Autodesk Fusion 360 part; units mm, degrees
(part 2 of 3)
  line L895 (-90.4101, 0.75) -> (-90.4101, -0.75)
  line L896 (-91.5158, -0.75) -> (-91.5158, 0.75)
  line L897 (-84.4232, -19.1686) -> (-85.7222, -18.4186)
  line L898 (-101.5213, 0.75) -> (-101.5213, -0.75)
  line L899 (-80.3306, -0.75) -> (-80.3306, 0.75)
  line L900 (-94.1139, 0.75) -> (-94.1139, -0.75)
  line L901 (-87.463, -11.6036) -> (-86.1639, -10.8536)
  line L902 (-81.6296, 1.5) -> (-82.9287, 0.75)
  line L903 (-100.2222, 1.5) -> (-101.5213, 0.75)
  line L904 (-121.5343, -20.6686) -> (-121.5343, -19.1686)
  line L905 (-97.8176, 0.75) -> (-97.8176, -0.75)
  line L906 (-72.6481, -11.6036) -> (-71.3491, -10.8536)
  line L907 (-85.3333, 1.5) -> (-86.6324, 0.75)
  line L908 (-63.1111, 1.5) -> (-64.4101, 0.75)
  line L909 (-122.299, -17.4932) -> (-121, -18.2432)
  line L910 (-95.2195, -0.75) -> (-95.2195, 0.75)
  line L911 (-84.0343, 0.75) -> (-85.3333, 1.5)
  line L912 (-96.5185, 1.5) -> (-97.8176, 0.75)
  line L913 (-70.2435, -10.8536) -> (-68.9444, -11.6036)
  line L914 (-80.3306, 0.75) -> (-81.6296, 1.5)
  line L915 (-76.6269, 0.75) -> (-77.9259, 1.5)
  line L916 (-59.3333, 1.5) -> (-60.6324, 0.75)
  line L917 (-40.8148, 1.5) -> (-42.1139, 0.75)
  line L918 (-51.6509, -10.8536) -> (-50.3519, -11.6036)
  line L919 (-107.3546, -10.8536) -> (-106.0556, -11.6036)
  line L920 (-46.9232, 0.75) -> (-48.2222, 1.5)
  line L921 (-55.6296, 1.5) -> (-56.9287, 0.75)
  line L922 (-61.8121, -0.75) -> (-61.8121, 0.75)
  line L923 (-48.2222, 1.5) -> (-49.5213, 0.75)
  line L924 (-64.4101, 0.75) -> (-64.4101, -0.75)
  line L925 (-50.6269, -0.75) -> (-50.6269, 0.75)
  line L926 (-69.2195, -0.75) -> (-69.2195, 0.75)
  line L927 (-62.762, -10.8536) -> (-61.463, -11.6036)
  line L928 (-71.8176, 0.75) -> (-71.8176, -0.75)
  line L929 (-117.8306, -19.1686) -> (-119.1296, -18.4186)
  line L930 (-120.4287, -20.6686) -> (-119.1296, -21.4186)
  line L931 (-122.299, -15.9932) -> (-122.299, -17.4932)
  line L932 (-119.1296, -21.4186) -> (-117.8306, -20.6686)
  line L933 (-106.3306, -0.75) -> (-106.3306, 0.75)
  line L934 (-119.701, -17.4932) -> (-119.701, -15.9932)
  line L935 (-53.225, 0.75) -> (-53.225, -0.75)
  line L936 (-117.8306, -20.6686) -> (-117.8306, -19.1686)
  line L937 (-120.4287, -19.1686) -> (-120.4287, -20.6686)
  line L938 (-54.3306, -0.75) -> (-54.3306, 0.75)
  line L939 (-109.7593, -11.6036) -> (-108.4602, -10.8536)
  line L940 (-92.8148, 1.5) -> (-94.1139, 0.75)
  line L941 (-68.9444, -11.6036) -> (-67.6454, -10.8536)
  line L942 (-37.1111, 1.5) -> (-38.4101, 0.75)
  line L943 (-98.6481, -11.6036) -> (-97.3491, -10.8536)
  line L944 (-98.9232, 0.75) -> (-100.2222, 1.5)
  line L945 (-87.8121, 0.75) -> (-89.1111, 1.5)
  line L946 (-95.2195, 0.75) -> (-96.5185, 1.5)
  line L947 (-39.5158, 0.75) -> (-40.8148, 1.5)
  line L948 (-92.4657, -10.8536) -> (-91.1667, -11.6036)
  line L949 (-54.3306, 0.75) -> (-55.6296, 1.5)
  line L950 (-83.7593, -11.6036) -> (-82.4602, -10.8536)
  line L951 (-91.5158, 0.75) -> (-92.8148, 1.5)
  line L952 (-44.5185, 1.5) -> (-45.8176, 0.75)
  line L953 (-94.9444, -11.6036) -> (-93.6454, -10.8536)
  line L954 (-99.9472, -10.8536) -> (-98.6481, -11.6036)
  line L955 (-87.0213, -20.6686) -> (-85.7222, -21.4186)
  line L956 (-73.9472, -10.8536) -> (-72.6481, -11.6036)
  line L957 (-89.1111, -1.5) -> (-87.8121, -0.75)
  line L958 (-47.9472, -10.8536) -> (-46.6481, -11.6036)
  line L959 (-70.5185, 1.5) -> (-71.8176, 0.75)
  line L960 (-50.6269, 0.75) -> (-51.9259, 1.5)
  line L961 (-77.6509, -10.8536) -> (-76.3519, -11.6036)
  line L962 (-35.8121, 0.75) -> (-37.1111, 1.5)
  line L963 (-66.8148, 1.5) -> (-68.1139, 0.75)
  line L964 (-79.6139, -19.1686) -> (-79.6139, -20.6686)
  line L965 (-66.4657, -10.8536) -> (-65.1667, -11.6036)
  line L966 (-44.2435, -10.8536) -> (-42.9444, -11.6036)
  line L967 (-72.9232, 0.75) -> (-74.2222, 1.5)
  line L968 (-107.6296, 1.5) -> (-108.9287, 0.75)
  line L969 (-54.0556, -11.6036) -> (-52.7565, -10.8536)
  line L970 (-91.1667, -11.6036) -> (-89.8676, -10.8536)
  line L971 (-65.1667, -11.6036) -> (-63.8676, -10.8536)
  line L972 (-77.0158, -19.1686) -> (-78.3148, -18.4186)
  line L973 (-84.4232, -20.6686) -> (-84.4232, -19.1686)
  line L974 (-61.8121, 0.75) -> (-63.1111, 1.5)
  line L975 (-74.2222, 1.5) -> (-75.5213, 0.75)
  line L976 (-58.0343, 0.75) -> (-59.3333, 1.5)
  line L977 (-69.2195, 0.75) -> (-70.5185, 1.5)
  line L978 (-51.9259, 1.5) -> (-53.225, 0.75)
  line L979 (-85.0583, -10.8536) -> (-83.7593, -11.6036)
  line L980 (-42.9444, -11.6036) -> (-41.6454, -10.8536)
  line L981 (-111.0583, -10.8536) -> (-109.7593, -11.6036)
  line L982 (-106.3306, 0.75) -> (-107.6296, 1.5)
  line L983 (-103.9259, 1.5) -> (-105.225, 0.75)
  line L984 (-50.3519, -11.6036) -> (-49.0528, -10.8536)
  line L985 (-57.7593, -11.6036) -> (-56.4602, -10.8536)
  line L986 (-43.2195, 0.75) -> (-44.5185, 1.5)
  line L987 (-102.6269, 0.75) -> (-103.9259, 1.5)
  line L988 (-55.3546, -10.8536) -> (-54.0556, -11.6036)
  line L989 (-76.3519, -11.6036) -> (-75.0528, -10.8536)
  line L990 (-78.3148, -18.4186) -> (-79.6139, -19.1686)
  line L991 (-106.0556, -11.6036) -> (-104.7565, -10.8536)
  line L992 (-88.762, -10.8536) -> (-87.463, -11.6036)
  line L993 (-103.6509, -10.8536) -> (-102.3519, -11.6036)
  line L994 (-59.0583, -10.8536) -> (-57.7593, -11.6036)
  line L995 (-89.1667, -8.1395) -> (-87.8676, -7.3895)
  line L996 (-65.5158, 0.75) -> (-66.8148, 1.5)
  line L997 (-96.2435, -10.8536) -> (-94.9444, -11.6036)
  line L998 (-77.9259, 1.5) -> (-79.225, 0.75)
  line L999 (-102.3519, -11.6036) -> (-101.0528, -10.8536)
  line L1000 (-80.0556, -11.6036) -> (-78.7565, -10.8536)
  line L1001 (-89.1111, 1.5) -> (-90.4101, 0.75)
  line L1002 (-46.6481, -11.6036) -> (-45.3491, -10.8536)
  line L1003 (-61.463, -11.6036) -> (-60.1639, -10.8536)
  line L1004 (-81.3546, -10.8536) -> (-80.0556, -11.6036)
  line L1005 (-96.299, -17.4932) -> (-95, -18.2432)
  line L1006 (-95, -15.2432) -> (-96.299, -15.9932)
  line L1007 (-83.3176, -20.6686) -> (-82.0185, -21.4186)
  line L1008 (-87.8676, -5.8895) -> (-89.1667, -5.1395)
  line L1009 (-99.0528, -5.8895) -> (-100.3519, -5.1395)
  line L1010 (-87.5926, -15.2432) -> (-88.8916, -15.9932)
  line L1011 (-179.9101, -19.1686) -> (-179.9101, -20.6686)
  line L1012 (-177.3121, -19.1686) -> (-178.6111, -18.4186)
  line L1013 (-173.5343, -19.1686) -> (-174.8333, -18.4186)
  line L1014 (-176.1324, -19.1686) -> (-176.1324, -20.6686)
  line L1015 (-173.5343, -20.6686) -> (-173.5343, -19.1686)
  line L1016 (-174.8333, -18.4186) -> (-176.1324, -19.1686)
  line L1017 (-178.6111, -21.4186) -> (-177.3121, -20.6686)
  line L1018 (-181.0158, -19.1686) -> (-182.3148, -18.4186)
  line L1019 (-184.7195, -19.1686) -> (-186.0185, -18.4186)
  line L1020 (-187.3176, -20.6686) -> (-186.0185, -21.4186)
  line L1021 (-188.4232, -19.1686) -> (-189.7222, -18.4186)
  line L1022 (-181.7805, -15.9932) -> (-181.7805, -17.4932)
  line L1023 (-180.8861, -12.5291) -> (-182.1852, -11.7791)
  line L1024 (-184.5899, -14.0291) -> (-184.5899, -12.5291)
  line L1025 (-186.5899, -15.9932) -> (-187.8889, -15.2432)
  line L1026 (-183.4842, -14.0291) -> (-182.1852, -14.7791)
  line L1027 (-184.1852, -15.2432) -> (-185.4842, -15.9932)
  line L1028 (-187.1879, -12.5291) -> (-187.1879, -14.0291)
  line L1029 (-183.4842, -12.5291) -> (-183.4842, -14.0291)
  line L1030 (-185.4842, -17.4932) -> (-184.1852, -18.2432)
  line L1031 (-185.8889, -11.7791) -> (-187.1879, -12.5291)
  line L1032 (-187.8889, -15.2432) -> (-189.1879, -15.9932)
  line L1033 (-166.1269, -20.6686) -> (-166.1269, -19.1686)
  line L1034 (-169.8306, -19.1686) -> (-171.1296, -18.4186)
  line L1035 (-171.1296, -21.4186) -> (-169.8306, -20.6686)
  line L1036 (-168.725, -20.6686) -> (-167.4259, -21.4186)
  line L1037 (-172.4287, -19.1686) -> (-172.4287, -20.6686)
  line L1038 (-172.4287, -20.6686) -> (-171.1296, -21.4186)
  line L1039 (-167.4259, -21.4186) -> (-166.1269, -20.6686)
  line L1040 (-168.725, -19.1686) -> (-168.725, -20.6686)
  line L1041 (-171.1296, -18.4186) -> (-172.4287, -19.1686)
  line L1042 (-167.4259, -18.4186) -> (-168.725, -19.1686)
  line L1043 (-179.9101, -20.6686) -> (-178.6111, -21.4186)
  line L1044 (-174.8333, -21.4186) -> (-173.5343, -20.6686)
  line L1045 (-177.3121, -20.6686) -> (-177.3121, -19.1686)
  line L1046 (-173.4787, -14.0291) -> (-173.4787, -12.5291)
  line L1047 (-174.7778, -11.7791) -> (-176.0768, -12.5291)
  line L1048 (-175.4787, -15.9932) -> (-176.7778, -15.2432)
  line L1049 (-179.1824, -15.9932) -> (-180.4815, -15.2432)
  line L1050 (-176.7778, -15.2432) -> (-178.0768, -15.9932)
  line L1051 (-174.7778, -14.7791) -> (-173.4787, -14.0291)
  line L1052 (-179.1824, -17.4932) -> (-179.1824, -15.9932)
  line L1053 (-173.4787, -12.5291) -> (-174.7778, -11.7791)
  line L1054 (-179.7805, -12.5291) -> (-179.7805, -14.0291)
  line L1055 (-176.7778, -18.2432) -> (-175.4787, -17.4932)
  line L1056 (-177.1824, -12.5291) -> (-178.4815, -11.7791)
  line L1057 (-178.4815, -14.7791) -> (-177.1824, -14.0291)
  line L1058 (-189.463, -8.1395) -> (-188.1639, -7.3895)
  line L1059 (-176.0768, -12.5291) -> (-176.0768, -14.0291)
  line L1060 (-182.1852, -14.7791) -> (-180.8861, -14.0291)
  line L1061 (-185.4842, -15.9932) -> (-185.4842, -17.4932)
  line L1062 (-182.8861, -17.4932) -> (-182.8861, -15.9932)
  line L1063 (-184.1852, -18.2432) -> (-182.8861, -17.4932)
  line L1064 (-182.1852, -11.7791) -> (-183.4842, -12.5291)
  line L1065 (-189.1879, -15.9932) -> (-189.1879, -17.4932)
  line L1066 (-189.1879, -17.4932) -> (-187.8889, -18.2432)
  line L1067 (-178.6111, -18.4186) -> (-179.9101, -19.1686)
  line L1068 (-176.1324, -20.6686) -> (-174.8333, -21.4186)
  line L1069 (-168.5953, -12.5291) -> (-168.5953, -14.0291)
  line L1070 (-169.701, -14.0291) -> (-169.701, -12.5291)
  line L1071 (-166.8916, -15.9932) -> (-166.8916, -17.4932)
  line L1072 (-169.2963, -18.2432) -> (-167.9973, -17.4932)
  line L1073 (-171, -11.7791) -> (-172.299, -12.5291)
  line L1074 (-167.9973, -15.9932) -> (-169.2963, -15.2432)
  line L1075 (-169.701, -12.5291) -> (-171, -11.7791)
  line L1076 (-170.5953, -15.9932) -> (-170.5953, -17.4932)
  line L1077 (-169.2963, -15.2432) -> (-170.5953, -15.9932)
  line L1078 (-172.299, -12.5291) -> (-172.299, -14.0291)
  line L1079 (-189.5926, -14.7791) -> (-188.2936, -14.0291)
  line L1080 (-167.2963, -11.7791) -> (-168.5953, -12.5291)
  line L1081 (-170.5953, -17.4932) -> (-169.2963, -18.2432)
  line L1082 (-173, -18.2432) -> (-171.701, -17.4932)
  line L1083 (-171.701, -17.4932) -> (-171.701, -15.9932)
  line L1084 (-189.7222, -21.4186) -> (-188.4232, -20.6686)
  line L1085 (-181.0158, -20.6686) -> (-181.0158, -19.1686)
  line L1086 (-182.3148, -18.4186) -> (-183.6139, -19.1686)
  line L1087 (-183.6139, -20.6686) -> (-182.3148, -21.4186)
  line L1088 (-187.3176, -19.1686) -> (-187.3176, -20.6686)
  line L1089 (-169.8306, -20.6686) -> (-169.8306, -19.1686)
  line L1090 (-166.1269, -19.1686) -> (-167.4259, -18.4186)
  line L1091 (-172.299, -14.0291) -> (-171, -14.7791)
  line L1092 (-167.9973, -17.4932) -> (-167.9973, -15.9932)
  line L1093 (-165.9973, -12.5291) -> (-167.2963, -11.7791)
  line L1094 (-171, -14.7791) -> (-169.701, -14.0291)
  line L1095 (-136.1639, -7.3895) -> (-136.1639, -5.8895)
  line L1096 (-167.8121, -4.2141) -> (-167.8121, -2.7141)
  line L1097 (-144.4657, -9.3536) -> (-144.4657, -10.8536)
  line L1098 (-135.6296, -1.9641) -> (-136.9287, -2.7141)
  line L1099 (-141.1111, -1.5) -> (-139.8121, -0.75)
  line L1100 (-171.5158, -2.7141) -> (-172.8148, -1.9641)
  line L1101 (-149.2195, -4.2141) -> (-149.2195, -2.7141)
  line L1102 (-151.0528, -5.8895) -> (-152.3519, -5.1395)
  line L1103 (-181.9259, -1.5) -> (-180.6269, -0.75)
  line L1104 (-130.0556, -8.1395) -> (-128.7565, -7.3895)
  line L1105 (-141.8121, -4.2141) -> (-141.8121, -2.7141)
  line L1106 (-134.9287, -0.75) -> (-133.6296, -1.5)
  line L1107 (-169.1111, -1.9641) -> (-170.4101, -2.7141)
  line L1108 (-123.3491, -10.8536) -> (-123.3491, -9.3536)
  line L1109 (-136.9287, -4.2141) -> (-135.6296, -4.9641)
  line L1110 (-183.225, -0.75) -> (-181.9259, -1.5)
  line L1111 (-151.8176, -4.2141) -> (-150.5185, -4.9641)
  line L1112 (-168.4657, -5.8895) -> (-168.4657, -7.3895)
  line L1113 (-146.8148, -4.9641) -> (-145.5158, -4.2141)
  line L1114 (-153.6509, -7.3895) -> (-152.3519, -8.1395)
  line L1115 (-130.0556, -5.1395) -> (-131.3546, -5.8895)
  line L1116 (-170.8148, -1.5) -> (-169.5158, -0.75)
  line L1117 (-120.8148, -1.9641) -> (-122.1139, -2.7141)
  line L1118 (-170.4657, -9.3536) -> (-170.4657, -10.8536)
  line L1119 (-152.9232, -4.2141) -> (-152.9232, -2.7141)
  line L1120 (-141.8676, -9.3536) -> (-143.1667, -8.6036)
  line L1121 (-149.2195, -2.7141) -> (-150.5185, -1.9641)
  line L1122 (-151.9472, -9.3536) -> (-151.9472, -10.8536)
  line L1123 (-131.9259, -1.9641) -> (-133.225, -2.7141)
  line L1124 (-132.4602, -5.8895) -> (-133.7593, -5.1395)
  line L1125 (-172.2435, -7.3895) -> (-170.9444, -8.1395)
  line L1126 (-152.3519, -8.1395) -> (-151.0528, -7.3895)
  line L1127 (-148.1139, -2.7141) -> (-148.1139, -4.2141)
  line L1128 (-122.2435, -9.3536) -> (-122.2435, -10.8536)
  line L1129 (-153.5213, -0.75) -> (-152.2222, -1.5)
  line L1130 (-168.4101, -0.75) -> (-167.1111, -1.5)
  line L1131 (-181.5213, -4.2141) -> (-180.2222, -4.9641)
  line L1132 (-154.2222, -4.9641) -> (-152.9232, -4.2141)
  line L1133 (-146.9444, -8.6036) -> (-148.2435, -9.3536)
  line L1134 (-182.6269, -4.2141) -> (-182.6269, -2.7141)
  line L1135 (-181.5213, -2.7141) -> (-181.5213, -4.2141)
  line L1136 (-149.3491, -9.3536) -> (-150.6481, -8.6036)
  line L1137 (-152.3519, -5.1395) -> (-153.6509, -5.8895)
  line L1138 (-137.3333, -1.5) -> (-136.0343, -0.75)
  line L1139 (-171.5158, -4.2141) -> (-171.5158, -2.7141)
  line L1140 (-155.5213, -4.2141) -> (-154.2222, -4.9641)
  line L1141 (-119.6454, -9.3536) -> (-120.9444, -8.6036)
  line L1142 (-143.1111, -4.9641) -> (-141.8121, -4.2141)
  line L1143 (-167.8676, -10.8536) -> (-167.8676, -9.3536)
  line L1144 (-133.225, -4.2141) -> (-131.9259, -4.9641)
  line L1145 (-134.4602, -10.8536) -> (-134.4602, -9.3536)
  line L1146 (-152.2222, -1.5) -> (-150.9232, -0.75)
  line L1147 (-119.5158, -2.7141) -> (-120.8148, -1.9641)
  line L1148 (-151.8176, -2.7141) -> (-151.8176, -4.2141)
  line L1149 (-154.2222, -1.9641) -> (-155.5213, -2.7141)
  line L1150 (-141.8121, -2.7141) -> (-143.1111, -1.9641)
  line L1151 (-125.9472, -9.3536) -> (-125.9472, -10.8536)
  line L1152 (-169.1111, -4.9641) -> (-167.8121, -4.2141)
  line L1153 (-143.1111, -1.9641) -> (-144.4101, -2.7141)
  line L1154 (-132.0556, -8.6036) -> (-133.3546, -9.3536)
  line L1155 (-151.0528, -7.3895) -> (-151.0528, -5.8895)
  line L1156 (-128.7565, -7.3895) -> (-128.7565, -5.8895)
  line L1157 (-172.1139, -0.75) -> (-170.8148, -1.5)
  line L1158 (-148.6481, -8.1395) -> (-147.3491, -7.3895)
  line L1159 (-127.9101, -20.6686) -> (-126.6111, -21.4186)
  line L1160 (-160.9287, -0.75) -> (-159.6296, -1.5)
  line L1161 (-156.3148, -21.4186) -> (-155.0158, -20.6686)
  line L1162 (-141.9973, -15.9932) -> (-143.2963, -15.2432)
  line L1163 (-166.8916, -17.4932) -> (-165.5926, -18.2432)
  line L1164 (-127.7805, -14.0291) -> (-126.4815, -14.7791)
  line L1165 (-161.8889, -15.2432) -> (-163.1879, -15.9932)
  line L1166 (-123.4787, -17.4932) -> (-123.4787, -15.9932)
  line L1167 (-138.762, -7.3895) -> (-137.463, -8.1395)
  line L1168 (-188.1639, -7.3895) -> (-188.1639, -5.8895)
  line L1169 (-161.6296, -4.9641) -> (-160.3306, -4.2141)
  line L1170 (-129.0158, -19.1686) -> (-130.3148, -18.4186)
  line L1171 (-187.7593, -8.6036) -> (-189.0583, -9.3536)
  line L1172 (-126.6111, -18.4186) -> (-127.9101, -19.1686)
  line L1173 (-185.3546, -9.3536) -> (-185.3546, -10.8536)
  line L1174 (-187.0583, -5.8895) -> (-187.0583, -7.3895)
  line L1175 (-156.8861, -17.4932) -> (-156.8861, -15.9932)
  line L1176 (-148.299, -17.4932) -> (-147, -18.2432)
  line L1177 (-128.4815, -15.2432) -> (-129.7805, -15.9932)
  line L1178 (-160.3306, -2.7141) -> (-161.6296, -1.9641)
  line L1179 (-139.9973, -12.5291) -> (-141.2963, -11.7791)
  line L1180 (-159.7593, -5.1395) -> (-161.0583, -5.8895)
  line L1181 (-138.2936, -17.4932) -> (-138.2936, -15.9932)
  line L1182 (-179.5213, -0.75) -> (-178.2222, -1.5)
  line L1183 (-138.6324, -0.75) -> (-137.3333, -1.5)
  line L1184 (-185.7593, -8.1395) -> (-184.4602, -7.3895)
  line L1185 (-131.6139, -19.1686) -> (-131.6139, -20.6686)
  line L1186 (-128.4815, -18.2432) -> (-127.1824, -17.4932)
  line L1187 (-156.1852, -14.7791) -> (-154.8861, -14.0291)
  line L1188 (-160.4602, -10.8536) -> (-160.4602, -9.3536)
  line L1189 (-163.0583, -9.3536) -> (-163.0583, -10.8536)
  line L1190 (-186.4602, -9.3536) -> (-187.7593, -8.6036)
  line L1191 (-155.7805, -17.4932) -> (-154.4815, -18.2432)
  line L1192 (-157.6139, -20.6686) -> (-156.3148, -21.4186)
  line L1193 (-139.0213, -20.6686) -> (-137.7222, -21.4186)
  line L1194 (-186.4602, -10.8536) -> (-186.4602, -9.3536)
  line L1195 (-124.0768, -12.5291) -> (-124.0768, -14.0291)
  line L1196 (-162.2936, -12.5291) -> (-163.5926, -11.7791)
  line L1197 (-142.725, -19.1686) -> (-142.725, -20.6686)
  line L1198 (-147.5343, -20.6686) -> (-147.5343, -19.1686)
  line L1199 (-130.3148, -18.4186) -> (-131.6139, -19.1686)
  line L1200 (-189.0583, -9.3536) -> (-189.0583, -10.8536)
  line L1201 (-161.0583, -7.3895) -> (-159.7593, -8.1395)
  line L1202 (-154.8861, -12.5291) -> (-156.1852, -11.7791)
  line L1203 (-130.1852, -11.7791) -> (-131.4842, -12.5291)
  line L1204 (-127.9101, -19.1686) -> (-127.9101, -20.6686)
  line L1205 (-126.4815, -11.7791) -> (-127.7805, -12.5291)
  line L1206 (-154.4815, -18.2432) -> (-153.1824, -17.4932)
  line L1207 (-162.9287, -2.7141) -> (-162.9287, -4.2141)
  line L1208 (-137.7222, -18.4186) -> (-139.0213, -19.1686)
  line L1209 (-187.0583, -7.3895) -> (-185.7593, -8.1395)
  line L1210 (-164.6324, -0.75) -> (-163.3333, -1.5)
  line L1211 (-128.8861, -14.0291) -> (-128.8861, -12.5291)
  line L1212 (-184.4602, -7.3895) -> (-184.4602, -5.8895)
  line L1213 (-149.4787, -17.4932) -> (-149.4787, -15.9932)
  line L1214 (-150.0768, -14.0291) -> (-148.7778, -14.7791)
  line L1215 (-154.8861, -14.0291) -> (-154.8861, -12.5291)
  line L1216 (-142.725, -20.6686) -> (-141.4259, -21.4186)
  line L1217 (-164.2936, -17.4932) -> (-164.2936, -15.9932)
  line L1218 (-156.7565, -9.3536) -> (-158.0556, -8.6036)
  line L1219 (-124.0768, -14.0291) -> (-122.7778, -14.7791)
  line L1220 (-166.762, -9.3536) -> (-166.762, -10.8536)
  line L1221 (-130.1852, -14.7791) -> (-128.8861, -14.0291)
  line L1222 (-149.4787, -15.9932) -> (-150.7778, -15.2432)
  line L1223 (-151.3121, -20.6686) -> (-151.3121, -19.1686)
  line L1224 (-157.3546, -5.8895) -> (-157.3546, -7.3895)
  line L1225 (-131.6139, -20.6686) -> (-130.3148, -21.4186)
  line L1226 (-148.8333, -21.4186) -> (-147.5343, -20.6686)
  line L1227 (-153.7805, -14.0291) -> (-152.4815, -14.7791)
  line L1228 (-159.4842, -17.4932) -> (-158.1852, -18.2432)
  line L1229 (-179.0528, -10.8536) -> (-179.0528, -9.3536)
  line L1230 (-163.5926, -11.7791) -> (-164.8916, -12.5291)
  line L1231 (-158.4602, -7.3895) -> (-158.4602, -5.8895)
  line L1232 (-121.4787, -14.0291) -> (-121.4787, -12.5291)
  line L1233 (-148.299, -15.9932) -> (-148.299, -17.4932)
  line L1234 (-157.4842, -12.5291) -> (-157.4842, -14.0291)
  line L1235 (-164.1639, -10.8536) -> (-164.1639, -9.3536)
  line L1236 (-125.1824, -14.0291) -> (-125.1824, -12.5291)
  line L1237 (-136.2936, -12.5291) -> (-137.5926, -11.7791)
  line L1238 (-178.3519, -8.1395) -> (-177.0528, -7.3895)
  line L1239 (-163.463, -8.1395) -> (-162.1639, -7.3895)
  line L1240 (-147.5343, -19.1686) -> (-148.8333, -18.4186)
  line L1241 (-162.1639, -5.8895) -> (-163.463, -5.1395)
  line L1242 (-136.4232, -19.1686) -> (-137.7222, -18.4186)
  line L1243 (-160.5899, -15.9932) -> (-161.8889, -15.2432)
  line L1244 (-130.3148, -21.4186) -> (-129.0158, -20.6686)
  line L1245 (-143.8306, -19.1686) -> (-145.1296, -18.4186)
  line L1246 (-162.1639, -7.3895) -> (-162.1639, -5.8895)
  line L1247 (-157.9259, -1.9641) -> (-159.225, -2.7141)
  line L1248 (-141.4259, -21.4186) -> (-140.1269, -20.6686)
  line L1249 (-150.7778, -15.2432) -> (-152.0768, -15.9932)
  line L1250 (-124.7778, -15.2432) -> (-126.0768, -15.9932)
  line L1251 (-134.0185, -21.4186) -> (-132.7195, -20.6686)
  line L1252 (-159.4842, -15.9932) -> (-159.4842, -17.4932)
  line L1253 (-155.5213, -2.7141) -> (-155.5213, -4.2141)
  line L1254 (-124.7778, -18.2432) -> (-123.4787, -17.4932)
  line L1255 (-159.7593, -8.1395) -> (-158.4602, -7.3895)
  line L1256 (-132.1852, -18.2432) -> (-130.8861, -17.4932)
  line L1257 (-143.2963, -15.2432) -> (-144.5953, -15.9932)
  line L1258 (-140.8916, -15.9932) -> (-140.8916, -17.4932)
  line L1259 (-130.8861, -15.9932) -> (-132.1852, -15.2432)
  line L1260 (-161.6296, -1.9641) -> (-162.9287, -2.7141)
  line L1261 (-147.4787, -14.0291) -> (-147.4787, -12.5291)
  line L1262 (-129.7805, -15.9932) -> (-129.7805, -17.4932)
  line L1263 (-143.8306, -20.6686) -> (-143.8306, -19.1686)
  line L1264 (-154.3519, -8.6036) -> (-155.6509, -9.3536)
  line L1265 (-135.8889, -18.2432) -> (-134.5899, -17.4932)
  line L1266 (-160.3306, -4.2141) -> (-160.3306, -2.7141)
  line L1267 (-180.7565, -7.3895) -> (-180.7565, -5.8895)
  line L1268 (-153.1824, -15.9932) -> (-154.4815, -15.2432)
  line L1269 (-166.6324, -4.2141) -> (-165.3333, -4.9641)
  line L1270 (-129.7805, -17.4932) -> (-128.4815, -18.2432)
  line L1271 (-143.2963, -18.2432) -> (-141.9973, -17.4932)
  line L1272 (-130.8861, -17.4932) -> (-130.8861, -15.9932)
  line L1273 (-122.7778, -11.7791) -> (-124.0768, -12.5291)
  line L1274 (-141.4259, -18.4186) -> (-142.725, -19.1686)
  line L1275 (-154.7565, -7.3895) -> (-154.7565, -5.8895)
  line L1276 (-133.8889, -14.7791) -> (-132.5899, -14.0291)
  line L1277 (-148.7778, -14.7791) -> (-147.4787, -14.0291)
  line L1278 (-143.701, -14.0291) -> (-143.701, -12.5291)
  line L1279 (-152.4815, -14.7791) -> (-151.1824, -14.0291)
  line L1280 (-183.3546, -7.3895) -> (-182.0556, -8.1395)
  line L1281 (-137.1879, -15.9932) -> (-137.1879, -17.4932)
  line L1282 (-127.7805, -12.5291) -> (-127.7805, -14.0291)
  line L1283 (-161.7593, -8.6036) -> (-163.0583, -9.3536)
  line L1284 (-126.0768, -17.4932) -> (-124.7778, -18.2432)
  line L1285 (-127.1824, -17.4932) -> (-127.1824, -15.9932)
  line L1286 (-158.0556, -8.6036) -> (-159.3546, -9.3536)
  line L1287 (-126.6111, -21.4186) -> (-125.3121, -20.6686)
  line L1288 (-180.3519, -8.6036) -> (-181.6509, -9.3536)
  line L1289 (-164.762, -5.8895) -> (-164.762, -7.3895)
  line L1290 (-126.4815, -14.7791) -> (-125.1824, -14.0291)
  line L1291 (-159.6296, -1.5) -> (-158.3306, -0.75)
  line L1292 (-151.1824, -12.5291) -> (-152.4815, -11.7791)
  line L1293 (-163.463, -5.1395) -> (-164.762, -5.8895)
  line L1294 (-157.3546, -7.3895) -> (-156.0556, -8.1395)
  line L1295 (-183.3546, -5.8895) -> (-183.3546, -7.3895)
  line L1296 (-139.5926, -18.2432) -> (-138.2936, -17.4932)
  line L1297 (-182.0556, -8.1395) -> (-180.7565, -7.3895)
  line L1298 (-145.701, -15.9932) -> (-147, -15.2432)
  line L1299 (-165.3333, -1.9641) -> (-166.6324, -2.7141)
  line L1300 (-163.5926, -14.7791) -> (-162.2936, -14.0291)
  line L1301 (-163.1879, -17.4932) -> (-161.8889, -18.2432)
  line L1302 (-128.8861, -12.5291) -> (-130.1852, -11.7791)
  line L1303 (-164.8916, -12.5291) -> (-164.8916, -14.0291)
  line L1304 (-157.225, -0.75) -> (-155.9259, -1.5)
  line L1305 (-134.5899, -15.9932) -> (-135.8889, -15.2432)
  line L1306 (-150.7778, -18.2432) -> (-149.4787, -17.4932)
  line L1307 (-134.0185, -18.4186) -> (-135.3176, -19.1686)
  line L1308 (-165.463, -8.6036) -> (-166.762, -9.3536)
  line L1309 (-156.0556, -5.1395) -> (-157.3546, -5.8895)
  line L1310 (-179.6509, -7.3895) -> (-178.3519, -8.1395)
  line L1311 (-157.9259, -4.9641) -> (-156.6269, -4.2141)
  line L1312 (-151.3121, -19.1686) -> (-152.6111, -18.4186)
  line L1313 (-161.1879, -12.5291) -> (-161.1879, -14.0291)
  line L1314 (-182.7565, -9.3536) -> (-184.0556, -8.6036)
  line L1315 (-161.8889, -18.2432) -> (-160.5899, -17.4932)
  line L1316 (-141.2963, -14.7791) -> (-139.9973, -14.0291)
  line L1317 (-147.4787, -12.5291) -> (-148.7778, -11.7791)
  line L1318 (-165.8676, -7.3895) -> (-165.8676, -5.8895)
  line L1319 (-135.3176, -19.1686) -> (-135.3176, -20.6686)
  line L1320 (-160.5899, -17.4932) -> (-160.5899, -15.9932)
  line L1321 (-123.4787, -15.9932) -> (-124.7778, -15.2432)
  line L1322 (-134.5899, -17.4932) -> (-134.5899, -15.9932)
  line L1323 (-165.5926, -18.2432) -> (-164.2936, -17.4932)
  line L1324 (-126.0768, -15.9932) -> (-126.0768, -17.4932)
  line L1325 (-153.9101, -20.6686) -> (-152.6111, -21.4186)
  line L1326 (-160.4602, -9.3536) -> (-161.7593, -8.6036)
  line L1327 (-158.4602, -5.8895) -> (-159.7593, -5.1395)
  line L1328 (-176.5185, -4.9641) -> (-175.2195, -4.2141)
  line L1329 (-179.6509, -5.8895) -> (-179.6509, -7.3895)
  line L1330 (-173.3491, -5.8895) -> (-174.6481, -5.1395)
  line L1331 (-184.0556, -8.6036) -> (-185.3546, -9.3536)
  line L1332 (-122.7778, -14.7791) -> (-121.4787, -14.0291)
  line L1333 (-154.4815, -15.2432) -> (-155.7805, -15.9932)
  line L1334 (-164.8916, -14.0291) -> (-163.5926, -14.7791)
  line L1335 (-179.0528, -9.3536) -> (-180.3519, -8.6036)
  line L1336 (-158.5899, -14.0291) -> (-158.5899, -12.5291)
  line L1337 (-151.1824, -14.0291) -> (-151.1824, -12.5291)
  line L1338 (-156.0556, -8.1395) -> (-154.7565, -7.3895)
  line L1339 (-181.6509, -9.3536) -> (-181.6509, -10.8536)
  line L1340 (-132.7195, -19.1686) -> (-134.0185, -18.4186)
  line L1341 (-163.3333, -1.5) -> (-162.0343, -0.75)
  line L1342 (-136.2936, -14.0291) -> (-136.2936, -12.5291)
  line L1343 (-135.1879, -12.5291) -> (-135.1879, -14.0291)
  line L1344 (-135.8889, -15.2432) -> (-137.1879, -15.9932)
  line L1345 (-155.6509, -9.3536) -> (-155.6509, -10.8536)
  line L1346 (-138.8916, -14.0291) -> (-137.5926, -14.7791)
  line L1347 (-145.1296, -18.4186) -> (-146.4287, -19.1686)
  line L1348 (-121.4787, -12.5291) -> (-122.7778, -11.7791)
  line L1349 (-129.0158, -20.6686) -> (-129.0158, -19.1686)
  line L1350 (-164.0343, -4.2141) -> (-164.0343, -2.7141)
  line L1351 (-125.1824, -12.5291) -> (-126.4815, -11.7791)
  line L1352 (-125.3121, -20.6686) -> (-125.3121, -19.1686)
  line L1353 (-131.4842, -12.5291) -> (-131.4842, -14.0291)
  line L1354 (-161.0583, -5.8895) -> (-161.0583, -7.3895)
  line L1355 (-131.4842, -14.0291) -> (-130.1852, -14.7791)
  line L1356 (-138.2936, -15.9932) -> (-139.5926, -15.2432)
  line L1357 (-145.701, -17.4932) -> (-145.701, -15.9932)
  line L1358 (-157.4842, -14.0291) -> (-156.1852, -14.7791)
  line L1359 (-146.4287, -20.6686) -> (-145.1296, -21.4186)
  line L1360 (-127.1824, -15.9932) -> (-128.4815, -15.2432)
  line L1361 (-164.0343, -2.7141) -> (-165.3333, -1.9641)
  line L1362 (-165.3333, -4.9641) -> (-164.0343, -4.2141)
  line L1363 (-159.8889, -14.7791) -> (-158.5899, -14.0291)
  line L1364 (-159.3546, -9.3536) -> (-159.3546, -10.8536)
  line L1365 (-125.3121, -19.1686) -> (-126.6111, -18.4186)
  line L1366 (-147, -18.2432) -> (-145.701, -17.4932)
  line L1367 (-182.7565, -10.8536) -> (-182.7565, -9.3536)
  line L1368 (-164.1639, -9.3536) -> (-165.463, -8.6036)
  line L1369 (-177.8176, -2.7141) -> (-177.8176, -4.2141)
  line L1370 (-159.225, -4.2141) -> (-157.9259, -4.9641)
  line L1371 (-161.1879, -14.0291) -> (-159.8889, -14.7791)
  line L1372 (-144.5953, -17.4932) -> (-143.2963, -18.2432)
  line L1373 (-150.0768, -12.5291) -> (-150.0768, -14.0291)
  line L1374 (-159.225, -2.7141) -> (-159.225, -4.2141)
  line L1375 (-174.1139, -2.7141) -> (-174.1139, -4.2141)
  line L1376 (-137.7222, -21.4186) -> (-136.4232, -20.6686)
  line L1377 (-163.1879, -15.9932) -> (-163.1879, -17.4932)
  line L1378 (-139.5926, -15.2432) -> (-140.8916, -15.9932)
  line L1379 (-152.4815, -11.7791) -> (-153.7805, -12.5291)
  line L1380 (-172.8148, -1.9641) -> (-174.1139, -2.7141)
  line L1381 (-164.762, -7.3895) -> (-163.463, -8.1395)
  line L1382 (-177.0528, -7.3895) -> (-177.0528, -5.8895)
  line L1383 (-148.7778, -11.7791) -> (-150.0768, -12.5291)
  line L1384 (-137.5926, -11.7791) -> (-138.8916, -12.5291)
  line L1385 (-152.0768, -17.4932) -> (-150.7778, -18.2432)
  line L1386 (-156.6269, -2.7141) -> (-157.9259, -1.9641)
  line L1387 (-184.4602, -5.8895) -> (-185.7593, -5.1395)
  line L1388 (-162.2936, -14.0291) -> (-162.2936, -12.5291)
  line L1389 (-178.2222, -1.5) -> (-176.9232, -0.75)
  line L1390 (-158.1852, -18.2432) -> (-156.8861, -17.4932)
  line L1391 (-177.8176, -4.2141) -> (-176.5185, -4.9641)
  line L1392 (-153.7805, -12.5291) -> (-153.7805, -14.0291)
  line L1393 (-156.6269, -4.2141) -> (-156.6269, -2.7141)
  line L1394 (-187.6296, -1.9641) -> (-188.9287, -2.7141)
  line L1395 (-164.2936, -15.9932) -> (-165.5926, -15.2432)
  line L1396 (-156.7565, -10.8536) -> (-156.7565, -9.3536)
  line L1397 (-145.1296, -21.4186) -> (-143.8306, -20.6686)
  line L1398 (-153.1824, -17.4932) -> (-153.1824, -15.9932)
  line L1399 (-159.8889, -11.7791) -> (-161.1879, -12.5291)
  line L1400 (-142.5953, -14.0291) -> (-141.2963, -14.7791)
  line L1401 (-150.1324, -19.1686) -> (-150.1324, -20.6686)
  line L1402 (-147, -15.2432) -> (-148.299, -15.9932)
  line L1403 (-132.5899, -14.0291) -> (-132.5899, -12.5291)
  line L1404 (-166.6324, -2.7141) -> (-166.6324, -4.2141)
  line L1405 (-152.0768, -15.9932) -> (-152.0768, -17.4932)
  line L1406 (-186.3306, -4.2141) -> (-186.3306, -2.7141)
  line L1407 (-135.3176, -20.6686) -> (-134.0185, -21.4186)
  line L1408 (-154.7565, -5.8895) -> (-156.0556, -5.1395)
  line L1409 (-155.7805, -15.9932) -> (-155.7805, -17.4932)
  line L1410 (-137.5926, -14.7791) -> (-136.2936, -14.0291)
  line L1411 (-145, -14.7791) -> (-143.701, -14.0291)
  line L1412 (-175.2195, -2.7141) -> (-176.5185, -1.9641)
  line L1413 (-146.299, -12.5291) -> (-146.299, -14.0291)
  line L1414 (-158.1852, -15.2432) -> (-159.4842, -15.9932)
  line L1415 (-146.299, -14.0291) -> (-145, -14.7791)
  line L1416 (-158.5899, -12.5291) -> (-159.8889, -11.7791)
  line L1417 (-155.9259, -1.5) -> (-154.6269, -0.75)
  line L1418 (-174.5185, -1.5) -> (-173.2195, -0.75)
  line L1419 (-152.6111, -21.4186) -> (-151.3121, -20.6686)
  line L1420 (-162.9287, -4.2141) -> (-161.6296, -4.9641)
  line L1421 (-133.4842, -17.4932) -> (-132.1852, -18.2432)
  line L1422 (-135.1879, -14.0291) -> (-133.8889, -14.7791)
  line L1423 (-175.2195, -4.2141) -> (-175.2195, -2.7141)
  line L1424 (-140.1269, -19.1686) -> (-141.4259, -18.4186)
  line L1425 (-141.9973, -17.4932) -> (-141.9973, -15.9932)
  line L1426 (-145, -11.7791) -> (-146.299, -12.5291)
  line L1427 (-139.9973, -14.0291) -> (-139.9973, -12.5291)
  line L1428 (-153.9101, -19.1686) -> (-153.9101, -20.6686)
  line L1429 (-139.0213, -19.1686) -> (-139.0213, -20.6686)
  line L1430 (-174.2435, -9.3536) -> (-174.2435, -10.8536)
  line L1431 (-156.1852, -11.7791) -> (-157.4842, -12.5291)
  line L1432 (-136.4232, -20.6686) -> (-136.4232, -19.1686)
  line L1433 (-152.6111, -18.4186) -> (-153.9101, -19.1686)
  line L1434 (-182.0556, -5.1395) -> (-183.3546, -5.8895)
  line L1435 (-146.4287, -19.1686) -> (-146.4287, -20.6686)
  line L1436 (-183.9259, -1.9641) -> (-185.225, -2.7141)
  line L1437 (-174.1139, -4.2141) -> (-172.8148, -4.9641)
  line L1438 (-137.463, -5.1395) -> (-138.762, -5.8895)
  line L1439 (-178.3519, -5.1395) -> (-179.6509, -5.8895)
  line L1440 (-140.8916, -17.4932) -> (-139.5926, -18.2432)
  line L1441 (-142.5953, -12.5291) -> (-142.5953, -14.0291)
  line L1442 (-178.9232, -4.2141) -> (-178.9232, -2.7141)
  line L1443 (-177.9472, -9.3536) -> (-177.9472, -10.8536)
  line L1444 (-180.2222, -4.9641) -> (-178.9232, -4.2141)
  line L1445 (-174.6481, -8.1395) -> (-173.3491, -7.3895)
  line L1446 (-122.1139, -4.2141) -> (-120.8148, -4.9641)
  line L1447 (-175.3491, -9.3536) -> (-176.6481, -8.6036)
  line L1448 (-132.7195, -20.6686) -> (-132.7195, -19.1686)
  line L1449 (-156.8861, -15.9932) -> (-158.1852, -15.2432)
  line L1450 (-138.8916, -12.5291) -> (-138.8916, -14.0291)
  line L1451 (-148.8333, -18.4186) -> (-150.1324, -19.1686)
  line L1452 (-132.5899, -12.5291) -> (-133.8889, -11.7791)
  line L1453 (-144.5953, -15.9932) -> (-144.5953, -17.4932)
  line L1454 (-180.7565, -5.8895) -> (-182.0556, -5.1395)
  line L1455 (-182.6269, -2.7141) -> (-183.9259, -1.9641)
  line L1456 (-183.9259, -4.9641) -> (-182.6269, -4.2141)
  line L1457 (-173.3491, -7.3895) -> (-173.3491, -5.8895)
  line L1458 (-188.9287, -2.7141) -> (-188.9287, -4.2141)
  line L1459 (-188.9287, -4.2141) -> (-187.6296, -4.9641)
  line L1460 (-175.3491, -10.8536) -> (-175.3491, -9.3536)
  line L1461 (-172.9444, -8.6036) -> (-174.2435, -9.3536)
  line L1462 (-132.1852, -15.2432) -> (-133.4842, -15.9932)
  line L1463 (-186.3306, -2.7141) -> (-187.6296, -1.9641)
  line L1464 (-126.3519, -5.1395) -> (-127.6509, -5.8895)
  line L1465 (-176.5185, -1.9641) -> (-177.8176, -2.7141)
  line L1466 (-175.9472, -5.8895) -> (-175.9472, -7.3895)
  line L1467 (-174.6481, -5.1395) -> (-175.9472, -5.8895)
  line L1468 (-127.6509, -7.3895) -> (-126.3519, -8.1395)
  line L1469 (-176.6481, -8.6036) -> (-177.9472, -9.3536)
  line L1470 (-185.225, -4.2141) -> (-183.9259, -4.9641)
  line L1471 (-148.6481, -5.1395) -> (-149.9472, -5.8895)
  line L1472 (-140.1269, -20.6686) -> (-140.1269, -19.1686)
  line L1473 (-186.9287, -0.75) -> (-185.6296, -1.5)
  line L1474 (-133.4842, -15.9932) -> (-133.4842, -17.4932)
  line L1475 (-127.5213, -0.75) -> (-126.2222, -1.5)
  line L1476 (-143.701, -12.5291) -> (-145, -11.7791)
  line L1477 (-175.8176, -0.75) -> (-174.5185, -1.5)
  line L1478 (-185.7593, -5.1395) -> (-187.0583, -5.8895)
  line L1479 (-133.8889, -11.7791) -> (-135.1879, -12.5291)
  line L1480 (-185.6296, -1.5) -> (-184.3306, -0.75)
  line L1481 (-175.9472, -7.3895) -> (-174.6481, -8.1395)
  line L1482 (-137.1879, -17.4932) -> (-135.8889, -18.2432)
  line L1483 (-185.225, -2.7141) -> (-185.225, -4.2141)
  line L1484 (-149.9472, -7.3895) -> (-148.6481, -8.1395)
  line L1485 (-150.1324, -20.6686) -> (-148.8333, -21.4186)
  line L1486 (-170.9444, -5.1395) -> (-172.2435, -5.8895)
  line L1487 (-141.2963, -11.7791) -> (-142.5953, -12.5291)
  line L1488 (-187.6296, -4.9641) -> (-186.3306, -4.2141)
  line L1489 (-149.8176, -0.75) -> (-148.5185, -1.5)
  line L1490 (-130.7565, -9.3536) -> (-132.0556, -8.6036)
  line L1491 (-178.9232, -2.7141) -> (-180.2222, -1.9641)
  line L1492 (-150.5185, -1.9641) -> (-151.8176, -2.7141)
  line L1493 (-169.6454, -5.8895) -> (-170.9444, -5.1395)
  line L1494 (-172.8148, -4.9641) -> (-171.5158, -4.2141)
  line L1495 (-153.0528, -9.3536) -> (-154.3519, -8.6036)
  line L1496 (-180.2222, -1.9641) -> (-181.5213, -2.7141)
  line L1497 (-180.4815, -18.2432) -> (-179.1824, -17.4932)
  line L1498 (-178.0768, -15.9932) -> (-178.0768, -17.4932)
  line L1499 (-175.4787, -17.4932) -> (-175.4787, -15.9932)
  line L1500 (-179.7805, -14.0291) -> (-178.4815, -14.7791)
  line L1501 (-176.0768, -14.0291) -> (-174.7778, -14.7791)
  line L1502 (-181.7805, -17.4932) -> (-180.4815, -18.2432)
  line L1503 (-180.4815, -15.2432) -> (-181.7805, -15.9932)
  line L1504 (-177.1824, -14.0291) -> (-177.1824, -12.5291)
  line L1505 (-174.299, -15.9932) -> (-174.299, -17.4932)
  line L1506 (-188.1639, -5.8895) -> (-189.463, -5.1395)
  line L1507 (-178.4815, -11.7791) -> (-179.7805, -12.5291)
  line L1508 (-178.0768, -17.4932) -> (-176.7778, -18.2432)
  line L1509 (-186.0185, -21.4186) -> (-184.7195, -20.6686)
  line L1510 (-182.3148, -21.4186) -> (-181.0158, -20.6686)
  line L1511 (-183.6139, -19.1686) -> (-183.6139, -20.6686)
  line L1512 (-186.0185, -18.4186) -> (-187.3176, -19.1686)
  line L1513 (-184.7195, -20.6686) -> (-184.7195, -19.1686)
  line L1514 (-189.3333, -1.5) -> (-188.0343, -0.75)
  line L1515 (-139.463, -8.6036) -> (-140.762, -9.3536)
  line L1516 (-167.1667, -5.1395) -> (-168.4657, -5.8895)
  line L1517 (-132.4602, -7.3895) -> (-132.4602, -5.8895)
  line L1518 (-148.5185, -1.5) -> (-147.2195, -0.75)
  line L1519 (-170.4101, -4.2141) -> (-169.1111, -4.9641)
  line L1520 (-170.9444, -8.1395) -> (-169.6454, -7.3895)
  line L1521 (-143.1667, -8.6036) -> (-144.4657, -9.3536)
  line L1522 (-129.9259, -1.5) -> (-128.6269, -0.75)
  line L1523 (-135.0583, -5.8895) -> (-135.0583, -7.3895)
  line L1524 (-144.9444, -5.1395) -> (-146.2435, -5.8895)
  line L1525 (-124.5185, -1.9641) -> (-125.8176, -2.7141)
  line L1526 (-125.0528, -5.8895) -> (-126.3519, -5.1395)
  line L1527 (-133.6296, -1.5) -> (-132.3306, -0.75)
  line L1528 (-169.1667, -8.6036) -> (-170.4657, -9.3536)
  line L1529 (-127.6509, -5.8895) -> (-127.6509, -7.3895)
  line L1530 (-123.9472, -5.8895) -> (-123.9472, -7.3895)
  line L1531 (-171.6454, -9.3536) -> (-172.9444, -8.6036)
  line L1532 (-129.5213, -4.2141) -> (-128.2222, -4.9641)
  line L1533 (-118.4101, -2.7141) -> (-118.4101, -4.2141)
  line L1534 (-118.9444, -8.1395) -> (-117.6454, -7.3895)
  line L1535 (-133.7593, -8.1395) -> (-132.4602, -7.3895)
  line L1536 (-172.2435, -5.8895) -> (-172.2435, -7.3895)
  line L1537 (-168.4657, -7.3895) -> (-167.1667, -8.1395)
  line L1538 (-134.3306, -2.7141) -> (-135.6296, -1.9641)
  line L1539 (-141.1667, -5.1395) -> (-142.4657, -5.8895)
  line L1540 (-120.9444, -8.6036) -> (-122.2435, -9.3536)
  line L1541 (-129.6509, -9.3536) -> (-129.6509, -10.8536)
  line L1542 (-115.8121, -2.7141) -> (-117.1111, -1.9641)
  line L1543 (-135.7593, -8.6036) -> (-137.0583, -9.3536)
  line L1544 (-130.6269, -2.7141) -> (-131.9259, -1.9641)
  line L1545 (-149.3491, -10.8536) -> (-149.3491, -9.3536)
  line L1546 (-124.5185, -4.9641) -> (-123.2195, -4.2141)
  line L1547 (-118.4101, -4.2141) -> (-117.1111, -4.9641)
  line L1548 (-143.6454, -7.3895) -> (-143.6454, -5.8895)
  line L1549 (-131.9259, -4.9641) -> (-130.6269, -4.2141)
  line L1550 (-123.2195, -2.7141) -> (-124.5185, -1.9641)
  line L1551 (-131.3546, -7.3895) -> (-130.0556, -8.1395)
  line L1552 (-153.0528, -10.8536) -> (-153.0528, -9.3536)
  line L1553 (-169.6454, -7.3895) -> (-169.6454, -5.8895)
  line L1554 (-150.5185, -4.9641) -> (-149.2195, -4.2141)
  line L1555 (-149.9472, -5.8895) -> (-149.9472, -7.3895)
  line L1556 (-143.6454, -5.8895) -> (-144.9444, -5.1395)
  line L1557 (-134.4602, -9.3536) -> (-135.7593, -8.6036)
  line L1558 (-123.2195, -4.2141) -> (-123.2195, -2.7141)
  line L1559 (-142.4101, -0.75) -> (-141.1111, -1.5)
  line L1560 (-139.3333, -1.9641) -> (-140.6324, -2.7141)
  line L1561 (-138.0343, -4.2141) -> (-138.0343, -2.7141)
  line L1562 (-153.6509, -5.8895) -> (-153.6509, -7.3895)
  line L1563 (-119.5158, -4.2141) -> (-119.5158, -2.7141)
  line L1564 (-121.3491, -7.3895) -> (-121.3491, -5.8895)
  line L1565 (-141.8676, -10.8536) -> (-141.8676, -9.3536)
  line L1566 (-147.3491, -7.3895) -> (-147.3491, -5.8895)
  line L1567 (-119.6454, -10.8536) -> (-119.6454, -9.3536)
  line L1568 (-128.2222, -1.9641) -> (-129.5213, -2.7141)
  line L1569 (-152.9232, -2.7141) -> (-154.2222, -1.9641)
  line L1570 (-145.5158, -2.7141) -> (-146.8148, -1.9641)
  line L1571 (-136.1639, -5.8895) -> (-137.463, -5.1395)
  line L1572 (-150.6481, -8.6036) -> (-151.9472, -9.3536)
  line L1573 (-140.6324, -4.2141) -> (-139.3333, -4.9641)
  line L1574 (-125.8176, -2.7141) -> (-125.8176, -4.2141)
  line L1575 (-171.6454, -10.8536) -> (-171.6454, -9.3536)
  line L1576 (-123.9472, -7.3895) -> (-122.6481, -8.1395)
  line L1577 (-136.9287, -2.7141) -> (-136.9287, -4.2141)
  line L1578 (-115.1111, -1.5) -> (-113.8121, -0.75)
  line L1579 (-122.6481, -5.1395) -> (-123.9472, -5.8895)
  line L1580 (-139.8676, -7.3895) -> (-139.8676, -5.8895)
  line L1581 (-122.6481, -8.1395) -> (-121.3491, -7.3895)
  line L1582 (-137.0583, -9.3536) -> (-137.0583, -10.8536)
  line L1583 (-126.2222, -1.5) -> (-124.9232, -0.75)
  line L1584 (-117.6454, -5.8895) -> (-118.9444, -5.1395)
  line L1585 (-116.4101, -0.75) -> (-115.1111, -1.5)
  line L1586 (-146.2435, -7.3895) -> (-144.9444, -8.1395)
  line L1587 (-138.1639, -10.8536) -> (-138.1639, -9.3536)
  line L1588 (-128.2222, -4.9641) -> (-126.9232, -4.2141)
  line L1589 (-133.225, -2.7141) -> (-133.225, -4.2141)
  line L1590 (-167.8121, -2.7141) -> (-169.1111, -1.9641)
  line L1591 (-170.4101, -2.7141) -> (-170.4101, -4.2141)
  line L1592 (-144.8148, -1.5) -> (-143.5158, -0.75)
  line L1593 (-146.8148, -1.9641) -> (-148.1139, -2.7141)
  line L1594 (-138.762, -5.8895) -> (-138.762, -7.3895)
  line L1595 (-141.1667, -8.1395) -> (-139.8676, -7.3895)
  line L1596 (-123.3491, -9.3536) -> (-124.6481, -8.6036)
  line L1597 (-144.4101, -4.2141) -> (-143.1111, -4.9641)
  line L1598 (-145.5158, -4.2141) -> (-145.5158, -2.7141)
  line L1599 (-121.3491, -5.8895) -> (-122.6481, -5.1395)
  line L1600 (-123.8176, -0.75) -> (-122.5185, -1.5)
  line L1601 (-117.1111, -1.9641) -> (-118.4101, -2.7141)
  line L1602 (-118.8148, -1.5) -> (-117.5158, -0.75)
  line L1603 (-128.3519, -8.6036) -> (-129.6509, -9.3536)
  line L1604 (-133.3546, -9.3536) -> (-133.3546, -10.8536)
  line L1605 (-128.7565, -5.8895) -> (-130.0556, -5.1395)
  line L1606 (-138.1639, -9.3536) -> (-139.463, -8.6036)
  line L1607 (-145.6454, -9.3536) -> (-146.9444, -8.6036)
  line L1608 (-137.463, -8.1395) -> (-136.1639, -7.3895)
  line L1609 (-130.7565, -10.8536) -> (-130.7565, -9.3536)
  line L1610 (-127.0528, -10.8536) -> (-127.0528, -9.3536)
  line L1611 (-138.0343, -2.7141) -> (-139.3333, -1.9641)
  line L1612 (-134.3306, -4.2141) -> (-134.3306, -2.7141)
  line L1613 (-142.4657, -7.3895) -> (-141.1667, -8.1395)
  line L1614 (-167.8676, -9.3536) -> (-169.1667, -8.6036)
  line L1615 (-135.6296, -4.9641) -> (-134.3306, -4.2141)
  line L1616 (-130.6269, -4.2141) -> (-130.6269, -2.7141)
  line L1617 (-140.6324, -2.7141) -> (-140.6324, -4.2141)
  line L1618 (-145.6454, -10.8536) -> (-145.6454, -9.3536)
  line L1619 (-117.6454, -7.3895) -> (-117.6454, -5.8895)
  line L1620 (-139.8676, -5.8895) -> (-141.1667, -5.1395)
  line L1621 (-122.5185, -1.5) -> (-121.2195, -0.75)
  line L1622 (-142.4657, -5.8895) -> (-142.4657, -7.3895)
  line L1623 (-125.0528, -7.3895) -> (-125.0528, -5.8895)
  line L1624 (-129.5213, -2.7141) -> (-129.5213, -4.2141)
  line L1625 (-120.2435, -5.8895) -> (-120.2435, -7.3895)
  line L1626 (-133.7593, -5.1395) -> (-135.0583, -5.8895)
  line L1627 (-126.9232, -4.2141) -> (-126.9232, -2.7141)
  line L1628 (-135.0583, -7.3895) -> (-133.7593, -8.1395)
  line L1629 (-148.2435, -9.3536) -> (-148.2435, -10.8536)
  line L1630 (-126.9232, -2.7141) -> (-128.2222, -1.9641)
  line L1631 (-131.225, -0.75) -> (-129.9259, -1.5)
  line L1632 (-120.2435, -7.3895) -> (-118.9444, -8.1395)
  line L1633 (-127.0528, -9.3536) -> (-128.3519, -8.6036)
  line L1634 (-139.3333, -4.9641) -> (-138.0343, -4.2141)
  line L1635 (-126.3519, -8.1395) -> (-125.0528, -7.3895)
  line L1636 (-131.3546, -5.8895) -> (-131.3546, -7.3895)
  line L1637 (-140.762, -9.3536) -> (-140.762, -10.8536)
  line L1638 (-147.3491, -5.8895) -> (-148.6481, -5.1395)
  line L1639 (-115.8121, -4.2141) -> (-115.8121, -2.7141)
  line L1640 (-125.8176, -4.2141) -> (-124.5185, -4.9641)
  line L1641 (-122.1139, -2.7141) -> (-122.1139, -4.2141)
  line L1642 (-146.1139, -0.75) -> (-144.8148, -1.5)
  line L1643 (-144.4101, -2.7141) -> (-144.4101, -4.2141)
  line L1644 (-146.2435, -5.8895) -> (-146.2435, -7.3895)
  line L1645 (-120.8148, -4.9641) -> (-119.5158, -4.2141)
  line L1646 (-118.9444, -5.1395) -> (-120.2435, -5.8895)
  line L1647 (-117.1111, -4.9641) -> (-115.8121, -4.2141)
  line L1648 (-120.1139, -0.75) -> (-118.8148, -1.5)
  line L1649 (-124.6481, -8.6036) -> (-125.9472, -9.3536)
  line L1650 (-148.1139, -4.2141) -> (-146.8148, -4.9641)
  line L1651 (-144.9444, -8.1395) -> (-143.6454, -7.3895)
  line L1652 (-184.5899, -12.5291) -> (-185.8889, -11.7791)
  line L1653 (-187.8889, -18.2432) -> (-186.5899, -17.4932)
  line L1654 (-186.5899, -17.4932) -> (-186.5899, -15.9932)
  line L1655 (-185.8889, -14.7791) -> (-184.5899, -14.0291)
  line L1656 (-187.1879, -14.0291) -> (-185.8889, -14.7791)
  line L1657 (-182.8861, -15.9932) -> (-184.1852, -15.2432)
  line L1658 (-188.2936, -14.0291) -> (-188.2936, -12.5291)
  line L1659 (-180.8861, -14.0291) -> (-180.8861, -12.5291)
  line L1660 (-188.4232, -20.6686) -> (-188.4232, -19.1686)
  line L1661 (-171.701, -15.9932) -> (-173, -15.2432)
  line L1662 (-165.9973, -14.0291) -> (-165.9973, -12.5291)
  line L1663 (-167.2963, -14.7791) -> (-165.9973, -14.0291)
  line L1664 (-188.2936, -12.5291) -> (-189.5926, -11.7791)
  line L1665 (-168.5953, -14.0291) -> (-167.2963, -14.7791)
  line L1666 (-186.9287, 0.75) -> (-186.9287, -0.75)
  line L1667 (-124.9232, -0.75) -> (-124.9232, 0.75)
  line L1668 (-134.9287, 0.75) -> (-134.9287, -0.75)
  line L1669 (-146.1139, 0.75) -> (-146.1139, -0.75)
  line L1670 (-136.0343, -0.75) -> (-136.0343, 0.75)
  line L1671 (-127.5213, 0.75) -> (-127.5213, -0.75)
  line L1672 (-138.6324, 0.75) -> (-138.6324, -0.75)
  line L1673 (-150.9232, -0.75) -> (-150.9232, 0.75)
  line L1674 (-161.3176, -19.1686) -> (-161.3176, -20.6686)
  line L1675 (-157.225, 0.75) -> (-157.225, -0.75)
  line L1676 (-163.7222, -21.4186) -> (-162.4232, -20.6686)
  line L1677 (-165.8121, -0.75) -> (-165.8121, 0.75)
  line L1678 (-155.0158, -20.6686) -> (-155.0158, -19.1686)
  line L1679 (-176.9232, -0.75) -> (-176.9232, 0.75)
  line L1680 (-180.6269, -0.75) -> (-180.6269, 0.75)
  line L1681 (-165.0213, -19.1686) -> (-165.0213, -20.6686)
  line L1682 (-160.0185, -18.4186) -> (-161.3176, -19.1686)
  line L1683 (-154.6269, -0.75) -> (-154.6269, 0.75)
  line L1684 (-116.4101, 0.75) -> (-116.4101, -0.75)
  line L1685 (-113.8121, -0.75) -> (-113.8121, 0.75)
  line L1686 (-117.5158, -0.75) -> (-117.5158, 0.75)
  line L1687 (-188.0343, -0.75) -> (-188.0343, 0)
  line L1688 (-123.8176, 0.75) -> (-123.8176, -0.75)
  line L1689 (-162.0343, -0.75) -> (-162.0343, 0.75)
  line L1690 (-160.0185, -21.4186) -> (-158.7195, -20.6686)
  line L1691 (-121.2195, -0.75) -> (-121.2195, 0.75)
  line L1692 (-160.9287, 0.75) -> (-160.9287, -0.75)
  line L1693 (-158.7195, -19.1686) -> (-160.0185, -18.4186)
  line L1694 (-153.5213, 0.75) -> (-153.5213, -0.75)
  line L1695 (-164.6324, 0.75) -> (-164.6324, -0.75)
  line L1696 (-183.225, 0.75) -> (-183.225, -0.75)
  line L1697 (-158.7195, -20.6686) -> (-158.7195, -19.1686)
  line L1698 (-163.7222, -18.4186) -> (-165.0213, -19.1686)
  line L1699 (-120.1139, 0.75) -> (-120.1139, -0.75)
  line L1700 (-143.5158, -0.75) -> (-143.5158, 0.75)
  line L1701 (-168.4101, 0.75) -> (-168.4101, -0.75)
  line L1702 (-169.5158, -0.75) -> (-169.5158, 0.75)
  line L1703 (-162.4232, -19.1686) -> (-163.7222, -18.4186)
  line L1704 (-179.5213, 0.75) -> (-179.5213, -0.75)
  line L1705 (-158.3306, -0.75) -> (-158.3306, 0.75)
  line L1706 (-172.1139, 0.75) -> (-172.1139, -0.75)
  line L1707 (-165.463, -11.6036) -> (-164.1639, -10.8536)
  line L1708 (-159.6296, 1.5) -> (-160.9287, 0.75)
  line L1709 (-178.2222, 1.5) -> (-179.5213, 0.75)
  line L1710 (-175.8176, 0.75) -> (-175.8176, -0.75)
  line L1711 (-150.6481, -11.6036) -> (-149.3491, -10.8536)
  line L1712 (-163.3333, 1.5) -> (-164.6324, 0.75)
  line L1713 (-141.1111, 1.5) -> (-142.4101, 0.75)
  line L1714 (-173.2195, -0.75) -> (-173.2195, 0.75)
  line L1715 (-162.0343, 0.75) -> (-163.3333, 1.5)
  line L1716 (-174.5185, 1.5) -> (-175.8176, 0.75)
  line L1717 (-148.2435, -10.8536) -> (-146.9444, -11.6036)
  line L1718 (-158.3306, 0.75) -> (-159.6296, 1.5)
  line L1719 (-154.6269, 0.75) -> (-155.9259, 1.5)
  line L1720 (-137.3333, 1.5) -> (-138.6324, 0.75)
  line L1721 (-118.8148, 1.5) -> (-120.1139, 0.75)
  line L1722 (-129.6509, -10.8536) -> (-128.3519, -11.6036)
  line L1723 (-185.3546, -10.8536) -> (-184.0556, -11.6036)
  line L1724 (-124.9232, 0.75) -> (-126.2222, 1.5)
  line L1725 (-133.6296, 1.5) -> (-134.9287, 0.75)
  line L1726 (-139.8121, -0.75) -> (-139.8121, 0.75)
  line L1727 (-126.2222, 1.5) -> (-127.5213, 0.75)
  line L1728 (-142.4101, 0.75) -> (-142.4101, -0.75)
  line L1729 (-128.6269, -0.75) -> (-128.6269, 0.75)
  line L1730 (-147.2195, -0.75) -> (-147.2195, 0.75)
  line L1731 (-140.762, -10.8536) -> (-139.463, -11.6036)
  line L1732 (-149.8176, 0.75) -> (-149.8176, -0.75)
  line L1733 (-184.3306, -0.75) -> (-184.3306, 0.75)
  line L1734 (-131.225, 0.75) -> (-131.225, -0.75)
  line L1735 (-132.3306, -0.75) -> (-132.3306, 0.75)
  line L1736 (-187.7593, -11.6036) -> (-186.4602, -10.8536)
  line L1737 (-170.8148, 1.5) -> (-172.1139, 0.75)
  line L1738 (-146.9444, -11.6036) -> (-145.6454, -10.8536)
  line L1739 (-115.1111, 1.5) -> (-116.4101, 0.75)
  line L1740 (-176.6481, -11.6036) -> (-175.3491, -10.8536)
  line L1741 (-176.9232, 0.75) -> (-178.2222, 1.5)
  line L1742 (-165.8121, 0.75) -> (-167.1111, 1.5)
  line L1743 (-173.2195, 0.75) -> (-174.5185, 1.5)
  line L1744 (-117.5158, 0.75) -> (-118.8148, 1.5)
  line L1745 (-170.4657, -10.8536) -> (-169.1667, -11.6036)
  line L1746 (-132.3306, 0.75) -> (-133.6296, 1.5)
  line L1747 (-161.7593, -11.6036) -> (-160.4602, -10.8536)
  line L1748 (-169.5158, 0.75) -> (-170.8148, 1.5)
  line L1749 (-122.5185, 1.5) -> (-123.8176, 0.75)
  line L1750 (-172.9444, -11.6036) -> (-171.6454, -10.8536)
  line L1751 (-177.9472, -10.8536) -> (-176.6481, -11.6036)
  line L1752 (-165.0213, -20.6686) -> (-163.7222, -21.4186)
  line L1753 (-151.9472, -10.8536) -> (-150.6481, -11.6036)
  line L1754 (-167.1111, -1.5) -> (-165.8121, -0.75)
  line L1755 (-125.9472, -10.8536) -> (-124.6481, -11.6036)
  line L1756 (-148.5185, 1.5) -> (-149.8176, 0.75)
  line L1757 (-128.6269, 0.75) -> (-129.9259, 1.5)
  line L1758 (-155.6509, -10.8536) -> (-154.3519, -11.6036)
  line L1759 (-113.8121, 0.75) -> (-115.1111, 1.5)
  line L1760 (-144.8148, 1.5) -> (-146.1139, 0.75)
  line L1761 (-157.6139, -19.1686) -> (-157.6139, -20.6686)
  line L1762 (-144.4657, -10.8536) -> (-143.1667, -11.6036)
  line L1763 (-122.2435, -10.8536) -> (-120.9444, -11.6036)
  line L1764 (-150.9232, 0.75) -> (-152.2222, 1.5)
  line L1765 (-185.6296, 1.5) -> (-186.9287, 0.75)